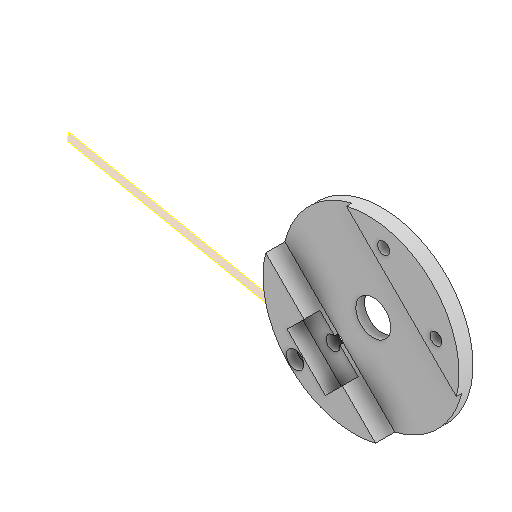
# Autodesk Inventor part: Matchboxscope_sample_v0
Saved by Autodesk Inventor 2022 (Build 260153000, 153)
## iProperties
Created: 2022-03-21
Part Number: Matchboxscope_sample_v0
Material: Generic
Document SubType Name: Modeling
Designer: Prakash Lab
Density: 1 g/cm^3
Appearance: Default
Author: Prakash Lab
Autodesk Inventor part; units mm, degrees
ref_plane "YZ Plane" through (0, 0, 0) normal (1, 0, 0) x (0, 1, 0)
ref_plane "XZ Plane" through (0, 0, 0) normal (0, 1, 0) x (-1, 0, 0)
ref_plane "XY Plane" through (0, 0, 0) normal (0, 0, 1) x (1, 0, 0)
ref_plane "Work Plane1" through (40.0005, 0, -24) normal (0, 0, 1) x (0.9792327, -0.2027397, 0)
sketch "Sketch1" plane through (40.0005, 0, -24) normal (0, 0, 1) x (0.9792327, -0.2027397, 0)
  circle A0 centre (8.0687, 11.3576) radius 25.9979 projected
  circle A1 centre (8.0703, 11.3562) radius 3.8103 projected
  circle A2 centre (8.0703, 11.3562) radius 5
  point P0 (-39.1698, -8.1097)
  dimension "d0" = 10
  constraints: 1 centre point, 1 coincident
  measures "d0" diameter of A2
extrude "Extrusion1" add sketch "Sketch1" along normal blind 4 contours A0
sketch "Sketch2" plane through (50.2043, 9.4859, -20) normal (0, 0, 1) x (1, 0, 0)
  line L0 (-50.2043, 54.0449) -> (-50.2043, -50.593) projected
  line L1 (-54.0467, -9.4859) -> (50.5907, -9.4859) projected
  line L2 (-15.9479, -15.1669) -> (4.4725, 20.2023)
  line L3 (4.4725, 20.2023) -> (19.4213, 5.2535)
  line L4 (19.4213, 5.2535) -> (-15.9479, -15.1669)
  line L5 (-39.0985, 39.0967) -> (35.6425, -35.6447)
  line L6 (-0.781, 0) -> (9.2905, 10.0715)
  line L7 (-0.781, 0) -> (13.4622, 0) construction
  line L8 (-15.9479, -15.1669) -> (-0.781, 0)
  circle A0 centre (4.4725, 20.2023) radius 1.6
  circle A1 centre (19.4213, 5.2535) radius 1.6
  circle A2 centre (-15.9479, -15.1669) radius 1.6 construction
  circle A3 centre (-16.8292, -16.048) radius 1.5
  dimension "d17" = 18
  dimension "d18" = 22
  dimension "d19" = 30
  dimension "d20" = 45
  dimension "d21" = 15
  dimension "d22" = 3.2
  dimension "d23" = 3.2
  dimension "d24" = 3.2
  dimension "d39" = 3
  constraints: 14 end point, 4 centre point, 3 coincident, 1 collinear, 1 equal length, 1 horizontal, 1 parallel, 3 other
  measures "d17" distance from line of L6.start L3
  measures "d18" distance from line of L5 L2.start
  measures "d19" angle of L2 L4
  measures "d20" angle of L7 L6
  measures "d21" angle of L2 L6
  measures "d22" diameter of A0
  measures "d23" diameter of A1
  measures "d24" diameter of A2
  measures "d39" diameter of A3
extrude "Extrusion2" cut sketch "Sketch2" against normal blind 3.4 contours A3 L8 L2 | L2 L4 A3 | A3 L4 L8 | A0 L3 L2 | L2 L3 A0 | A1 L3 L4 | L4 L3 A1
sketch "Sketch3" plane through (50.2043, 9.4859, -20) normal (0, 0, 1) x (1, 0, 0)
  line L0 (-35.7047, 22.4019) -> (13.1872, -35.1292) projected
  line L1 (32.542, -18.6808) -> (-16.3499, 38.8503) projected
  line L2 (40.2702, -21.1784) -> (-21.1782, 40.2703)
  line L3 (-21.1782, 40.2703) -> (-40.2702, 21.1784)
  line L4 (-40.2702, 21.1784) -> (21.1782, -40.2703)
  line L5 (21.1782, -40.2703) -> (40.2702, -21.1784)
  line L6 (40.2702, -21.1784) -> (-40.2702, 21.1784) construction
  line L7 (-21.1782, 40.2703) -> (21.1782, -40.2703) construction
  point P0 (0, 0)
  dimension "d16" = 27
  constraints: 12 end point, 2 midpoint, 2 parallel, 1 perpendicular
  measures "d16" distance of L3.end L2.end
extrude "Extrusion3" cut sketch "Sketch3" against normal blind 1.5
sketch "Sketch4" plane through (40.0005, 0, -20) normal (0, 0, 1) x (0.9792327, -0.2027397, 0)
  circle A0 centre (0.0169, -1.5448) radius 2 projected
extrude "Extrusion4" cut sketch "Sketch4" against normal blind 25.4
sketch "Sketch6" plane through (40.0005, 0, -20) normal (0, 0, 1) x (0.9792327, -0.2027397, 0)
  line L0 (-28.7292, -8.8539) -> (-25.804, -10.7757) projected
  line L1 (-20.2187, 4.1006) -> (-28.7292, -8.8539) projected
  line L2 (-20.2187, 4.1006) -> (-17.2935, 2.1789) projected
  circle A0 centre (-5.1575, -7.7691) radius 1.5 projected
  line L3 (0.0784, 0.4542) -> (-17.9131, 12.2738) projected
  arc A1 (-17.9131, 12.2738) -> (19.2256, -12.1245) centre (8.0687, 11.3576) ccw projected
  line L4 (-28.7292, -8.8539) -> (-20.2187, 4.1006)
  line L5 (-20.2187, 4.1006) -> (-38.152, 15.8819)
  line L6 (-38.152, 15.8819) -> (-46.6625, 2.9274)
  line L7 (-46.6625, 2.9274) -> (-28.7292, -8.8539)
  line L8 (-52.6907, 6.8876) -> (-44.1802, 19.8422)
  line L9 (-44.1802, 19.8422) -> (-14.4793, 0.3302)
  line L10 (-37.9848, 15.7721) -> (-46.4954, 2.8175)
  line L11 (-46.4954, 2.8175) -> (-42228058.7251, 27741750.4831)
  line L12 (-42228058.7251, 27741750.4831) -> (-52.6907, 6.8876)
  line L13 (-14.4793, 0.3302) -> (-37.9848, 15.7721)
  circle A2 centre (-5.1575, -7.7691) radius 1.5 projected
  circle A3 centre (-5.1575, -7.7691) radius 1.7
  circle A4 centre (26.0215, 20.4395) radius 2.75 projected
  circle A5 centre (8.3525, 32.0472) radius 2.45 projected
  circle A6 centre (26.0215, 20.4395) radius 1.6
  circle A7 centre (8.3525, 32.0472) radius 1.6
  arc A8 (0.0784, 0.4542) -> (1.8272, -0.6947) centre (0.0169, -1.5448) ccw projected
  line L14 (19.2256, -12.1245) -> (1.8272, -0.6947) projected
  point P0 (-39.1698, -8.1097)
  point P1 (8.0213, -4.7639)
  point P2 (-4.9332, 3.7467)
  dimension "d44" = 0
  dimension "d47" = 0
  dimension "d48" = 3.4
  dimension "d49" = 3.2
  dimension "d50" = 3.2
  constraints: 20 end point, 7 parallel, 3 centre point, 3 coincident, 3 perpendicular, 1 point on line
  measures "d44" distance between parallel lines of L7 L11
  measures "d47" distance between parallel lines of L2 L9
  measures "d48" diameter of A3
  measures "d49" diameter of A6
  measures "d50" diameter of A7
extrude "Extrusion6" add sketch "Sketch6" along normal blind 4 contours A8 L14 A1 L3 | A3
sketch "Sketch7" plane through (40.0005, 0, -16) normal (0, 0, 1) x (0.9792327, -0.2027397, 0)
  circle A0 centre (-5.1575, -7.7691) radius 2.45 projected
  circle A1 centre (8.3525, 32.0472) radius 2.75 projected
  circle A2 centre (26.0215, 20.4395) radius 2.75 projected
  point P0 (-39.1698, -8.1097)
hole "Hole1" at (69.6255, 14.7395, -16) at (54.6768, 29.6883, -16) at (33.375, -6.5621, -16) direction (0, 0, -1) diameter 3.4 end through all counterbore diameter 5 counterbore depth 3
sketch "Sketch8" plane through (40.0005, 0, -16) normal (0, 0, 1) x (0.9792327, -0.2027397, 0)
  line L0 (6.1726, -7.578) -> (16.7858, 8.5772) projected
  line L1 (16.7858, 8.5772) -> (3.8312, 17.0877) projected
  line L2 (-6.782, 0.9325) -> (3.8312, 17.0877) projected
  line L3 (6.1726, -7.578) -> (-6.782, 0.9325) projected
  line L4 (4.2509, -10.5033) -> (-8.7037, -1.9927) projected
  line L5 (4.2509, -10.5033) -> (6.1726, -7.578) projected
  line L6 (-8.7037, -1.9927) -> (-6.782, 0.9325) projected
  line L7 (4.2509, -10.5033) -> (-8.7037, -1.9927)
  line L8 (-8.7037, -1.9927) -> (-1.4754, 9.0101)
  line L9 (-1.4754, 9.0101) -> (11.4792, 0.4996)
  line L10 (11.4792, 0.4996) -> (4.2509, -10.5033)
  point P0 (-39.1698, -8.1097)
  point P1 (11.4792, 0.4996)
  point P2 (-1.4754, 9.0101)
  constraints: 8 end point, 3 equal length, 1 perpendicular
ref_plane "Work Plane2" through (12.9398, -24.5988, -20.5) normal (0, 0, 1) x (0.7071087, 0.7071049, 0)
extrude "Extrusion7" cut sketch "Sketch8" against normal up to surface (4.5 mm away) contours L3 L2 L9 L0 | L5 L4 L6 L3
body "Solid1"
